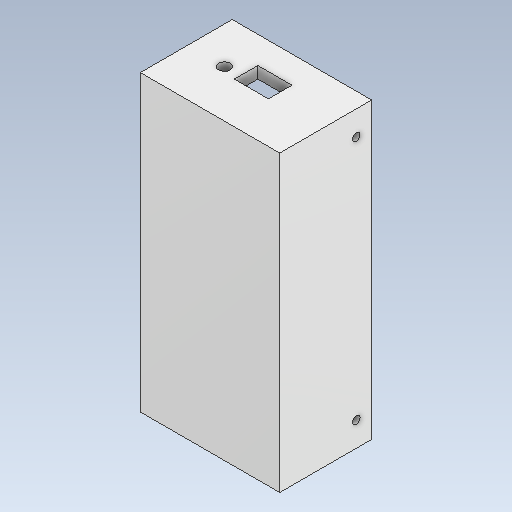
# Autodesk Inventor part: SENSOR_BOTTOM
Saved by Autodesk Inventor 2020 (Build 240168000, 168)
## iProperties
Created: 2023-03-28
Part Number: SENSOR_BOTTOM
Material: PC/ABS Plastic
Document SubType Name: Modeling
Designer: catsm
Density: 0.357273 g/cm^3
Appearance: Smooth - White
Author: catsm
Autodesk Inventor part; units mm, degrees
ref_plane "YZ Plane" through (0, 0, 0) normal (1, 0, 0) x (0, 1, 0)
ref_plane "XZ Plane" through (0, 0, 0) normal (0, 1, 0) x (-1, 0, 0)
ref_plane "Work Plane1" through (0, 0, 6.35) normal (0, 0, 1) x (1, 0, 0)
sketch "Sketch1" plane through (0, 0, 6.35) normal (0, 0, 1) x (1, 0, 0)
  line L0 (14.9733, -35.8014) -> (14.9733, 35.8014) projected
  line L1 (14.9733, 35.8014) -> (-14.9733, 35.8014) projected
  line L2 (-14.9733, 35.8014) -> (-14.9733, -35.8014) projected
  line L3 (-14.9733, -35.8014) -> (14.9733, -35.8014) projected
  circle A0 centre (-13.81, -28.5989) radius 0.6 projected
  circle A1 centre (-11.557, -24.257) radius 0.1524 projected
  circle A2 centre (-9.271, -23.749) radius 0.1524 projected
  circle A3 centre (-8.636, -22.606) radius 0.1524 projected
  circle A4 centre (-8.636, -19.939) radius 0.1524 projected
  circle A5 centre (-6.731, -35.3061) radius 0.1524 projected
  circle A6 centre (-5.842, -34.1631) radius 0.1524 projected
  circle A7 centre (-7.239, -31.8771) radius 0.1524 projected
  circle A8 centre (-5.08, -31.7501) radius 0.1524 projected
  circle A9 centre (-5.08, -30.8611) radius 0.1524 projected
  circle A10 centre (-1.016, -32.6391) radius 0.1524 projected
  circle A11 centre (-1.905, -27.9401) radius 0.1524 projected
  circle A12 centre (-4.318, -24.892) radius 0.1524 projected
  circle A13 centre (-5.842, -19.05) radius 0.1524 projected
  circle A14 centre (-5.08, -21.463) radius 0.1524 projected
  circle A15 centre (-5.08, -18.415) radius 0.1524 projected
  circle A16 centre (-4.191, -19.939) radius 0.1524 projected
  circle A17 centre (-4.191, -18.415) radius 0.1524 projected
  circle A18 centre (-11.176, -17.526) radius 0.1525 projected
  circle A19 centre (-13.014, -12.8141) radius 1.016 projected
  circle A20 centre (-7.874, -8.382) radius 1.85 projected
  circle A21 centre (-4.826, -17.526) radius 0.1524 projected
  circle A22 centre (-4.572, -5.715) radius 0.1524 projected
  circle A23 centre (-2.413, -6.35) radius 0.1524 projected
  circle A24 centre (-1.016, -5.715) radius 0.1524 projected
  circle A25 centre (4.953, -31.4961) radius 0.1524 projected
  circle A26 centre (6.35, -30.6071) radius 0.1524 projected
  circle A27 centre (6.19, -28.5989) radius 0.85 projected
  circle A28 centre (0.254, -24.638) radius 0.1524 projected
  circle A29 centre (1.27, -21.082) radius 0.1524 projected
  circle A30 centre (6.604, -26.2891) radius 0.1524 projected
  circle A31 centre (5.461, -21.717) radius 0.1524 projected
  circle A32 centre (8.509, -32.7661) radius 0.1524 projected
  circle A33 centre (8.636, -30.6071) radius 0.1524 projected
  circle A34 centre (12.986, -33.8141) radius 1.016 projected
  circle A35 centre (13.843, -30.0991) radius 0.1524 projected
  circle A36 centre (9.017, -24.892) radius 0.1524 projected
  circle A37 centre (9.779, -22.86) radius 0.1524 projected
  circle A38 centre (7.366, -21.717) radius 0.1524 projected
  circle A39 centre (-0.014, -16.637) radius 0.255 projected
  circle A40 centre (3.429, -7.62) radius 0.1524 projected
  circle A41 centre (10.287, -16.9782) radius 0.1524 projected
  circle A42 centre (10.033, -9.779) radius 0.1524 projected
  circle A43 centre (13.843, -17.526) radius 0.1524 projected
  circle A44 centre (-4.953, 11.303) radius 0.1524 projected
  circle A45 centre (-13.014, 33.886) radius 1.016 projected
  circle A46 centre (-3.8002, 24.494) radius 0.5 projected
  circle A47 centre (-4.4502, 34.2441) radius 0.5 projected
  circle A48 centre (-1.4001, 27.0939) radius 0.45 projected
  circle A49 centre (0, 13.843) radius 0.1524 projected
  circle A50 centre (3.8002, 24.494) radius 0.5 projected
  circle A51 centre (1.4001, 27.0939) radius 0.45 projected
  circle A52 centre (4.4502, 34.2441) radius 0.5 projected
  circle A53 centre (12.986, 33.886) radius 1.016 projected
  line L4 (-18.7833, -39.6114) -> (-18.7833, 39.6114)
  line L5 (-18.7833, 39.6114) -> (18.7833, 39.6114)
  line L6 (18.7833, 39.6114) -> (18.7833, -39.6114)
  line L7 (18.7833, -39.6114) -> (-18.7833, -39.6114)
  point P0 (0, 0)
  dimension "d1" = 3.81
  constraints: 8 end point, 3 other
  measures "d1" distance between parallel lines of L2 L4
extrude "Extrusion1" add sketch "Sketch1" along normal blind 3.175 contours L3 L2 L1 L0 | A0 | A1 | A2 | A3 | A4 | A5 | A6 | A7 | A8 | A9 | A10 | A11 | A12 | A13 | A14 | A15 | A16 | A17 | A18 | A19 | A20 | A21 | A22 | A23 | A24 | A25 | A26 | A27 | A28 | A29 | A30 | A31 | A32 | A33 | A34 | A35 | A36 | A37 | A38 | A39 | A40 | A41 | A42 | A43 | A44 | A45 | A46 | A47 | A48 | A49 | A50 | A51 | A52 | A53 | L4 L5 L6 L7
sketch "Sketch2" plane through (0, 0, 6.35) normal (0, 0, -1) x (-1, 0, 0)
  circle A0 centre (-12.986, -33.8141) radius 1.016 projected
  circle A1 centre (-12.986, 33.886) radius 1.016 projected
  circle A2 centre (13.014, 33.886) radius 1.016 projected
  circle A3 centre (-12.986, -33.8141) radius 3.556
  circle A4 centre (-12.986, 33.886) radius 3.556
  circle A5 centre (13.014, 33.886) radius 3.556
  line L0 (-12.986, 33.886) -> (13.014, 33.886)
  line L1 (13.014, 33.886) -> (13.014, -33.8141)
  line L2 (13.014, -33.8141) -> (-12.986, -33.8141)
  line L3 (-12.986, -33.8141) -> (-12.986, 33.886)
  circle A6 centre (13.014, -12.8141) radius 1.016
  circle A7 centre (13.014, -12.8141) radius 3.556
  point P0 (0, 0)
  dimension "d4" = 7.112
  dimension "d5" = 7.112
  dimension "d6" = 7.112
  dimension "d32" = 7.112
  constraints: 8 end point, 5 centre point, 4 coincident, 2 parallel, 1 horizontal, 1 perpendicular, 2 other
  measures "d4" diameter of A3
  measures "d5" diameter of A4
  measures "d6" diameter of A5
  measures "d32" diameter of A7
ref_plane "Work Plane2" through (-14.9733, -35.8014, 0) normal (0, 0, 1) x (1, 0, 0)
extrude "Extrusion2" add sketch "Sketch2" along normal up to surface (6.35 mm away) contours L2 L3 A0 | L2 A3 L3 A0 | A0 L3 A3 L2 | A0 L3 L2 | L3 A1 L0 A4 | A4 L0 A1 L3 | A7 L1 A6 | L1 A6 A7 | L3 L0 A1 | A1 L0 L3 | A6 L1 | L1 A6 | L0 A2 L1 A5 | A5 L1 A2 L0 | L0 L1 A2 | A2 L1 L0
sketch "Sketch3" plane through (12.986, -33.8141, 0) normal (0, 0, -1) x (-1, 0, 0)
  circle A0 centre (0, 67.7) radius 1.016 projected
  circle A1 centre (0, 0) radius 1.016 projected
  circle A2 centre (26, 67.7) radius 1.016 projected
  circle A3 centre (26, 21) radius 3.556 projected
  point P0 (12.986, 33.8141)
  constraints: 4 coincident
hole "Hole1" at (12.986, -33.8141, 0) at (12.986, 33.886, 0) at (-13.014, 33.886, 0) at (-13.014, -12.8141, 0) direction (0, 0, 1) diameter 3.556 depth 6.35 countersink diameter 3.81 countersink angle 82
sketch "Sketch4" plane through (0, 0, 6.35) normal (0, 0, -1) x (-1, 0, 0)
  circle A0 centre (-12.986, 33.886) radius 3.556 projected
  circle A1 centre (13.014, 33.886) radius 3.556 projected
  circle A2 centre (-12.986, -33.8141) radius 3.556 projected
  line L0 (18.7833, -39.6114) -> (-18.7833, -39.6114) projected
  line L1 (18.7833, 39.6114) -> (18.7833, -39.6114) projected
  line L2 (-18.7833, 39.6114) -> (18.7833, 39.6114) projected
  line L3 (-18.7833, -39.6114) -> (-18.7833, 39.6114) projected
  line L4 (-15.6083, 36.4364) -> (15.6083, 36.4364)
  line L5 (15.6083, 36.4364) -> (15.6083, -36.4364)
  line L6 (15.6083, -36.4364) -> (-15.6083, -36.4364)
  line L7 (-15.6083, -36.4364) -> (-15.6083, 36.4364)
  point P0 (0, 0)
  dimension "d17" = 3.175
  constraints: 8 end point, 3 other
  measures "d17" distance between parallel lines of L3 L7
extrude "Extrusion3" add sketch "Sketch4" along normal blind 21.59 contours L4 A0 | A0 L7 | A1 L4 | L7 A2 | L5 A1 | A2 L6 | L0 L3 L2 L1
sketch "Sketch5" plane through (-18.7833, 39.6114, 9.525) normal (0, 1, 0) x (1, 0, 0)
  line L0 (14.1836, 11.2166) -> (14.1836, 14.2664) projected
  line L1 (23.3831, 14.2664) -> (23.3831, 11.2166) projected
  line L2 (33.7567, 9.525) -> (33.7567, 11.125) projected
  line L3 (33.7567, 11.125) -> (3.81, 11.125) projected
  line L4 (3.81, 9.525) -> (3.81, 11.125) projected
  line L5 (33.7567, 9.525) -> (3.81, 9.525) projected
  line L6 (14.1836, 11.125) -> (23.3831, 11.125)
  line L7 (23.3831, 11.125) -> (23.3831, 17.475)
  line L8 (23.3831, 17.475) -> (14.1836, 17.475)
  line L9 (14.1836, 17.475) -> (14.1836, 11.125)
  point P0 (18.7833, 9.525)
  dimension "d20" = 6.35
  constraints: 8 end point, 2 parallel, 2 point on line, 1 horizontal, 1 perpendicular
  measures "d20" distance of L7.end L6.end
extrude "Extrusion4" cut sketch "Sketch5" against normal up to surface (3.175 mm away) contours L0 L9 L8 L7 L1 L3
sketch "Sketch6" plane through (-18.7833, 39.6114, 9.525) normal (0, 1, 0) x (1, 0, 0)
  circle A0 centre (9.9291, 12.7125) radius 1.5875
  line L0 (14.1836, 11.125) -> (14.1836, 17.475) projected
  line L1 (23.3831, 11.125) -> (14.1836, 11.125) projected
  point P0 (18.7833, 9.525)
  dimension "d23" = 4.2545
  dimension "d24" = 3.175
  dimension "d25" = 1.5875
  constraints: 1 centre point
  measures "d23" distance from line of L0 A0.centre
  measures "d24" diameter of A0
  measures "d25" distance from line of L1 A0.centre
extrude "Extrusion5" cut sketch "Sketch6" against normal up to surface (3.175 mm away)
sketch "Sketch7" plane through (18.7833, -39.6114, 9.525) normal (1, 0, 0) x (0, 0, -1)
  circle A0 centre (20.6375, 72.6187) radius 1.905 projected
  circle A1 centre (20.6375, 6.604) radius 1.778 projected
  circle A2 centre (20.6375, 6.604) radius 1.905 projected
  circle A3 centre (20.6375, 72.6187) radius 1.778 projected
  circle A4 centre (20.6375, 72.6187) radius 1.016
  circle A5 centre (20.6375, 6.604) radius 1.016
  point P0 (9.525, 39.6114)
  dimension "d33" = 2.032
  dimension "d34" = 2.032
  constraints: 2 centre point, 2 coincident
  measures "d33" diameter of A4
  measures "d34" diameter of A5
extrude "Extrusion6" cut sketch "Sketch7" against normal up to surface (37.5667 mm away) contours A4 | A5
body "Solid1"
